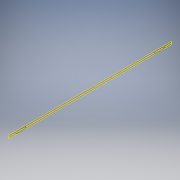
# Autodesk Inventor part: CentralLine
Saved by Autodesk Inventor 2016 (Build 200138000, 138)
## iProperties
Created: 2016-01-20
Part Number: CentralLine
Material: Generic
Document SubType Name: Modeling
Designer: KA ROSIE
Density: 1 g/cm^3
Appearance: Default
Author: KA ROSIE
Autodesk Inventor part; units mm, degrees
ref_plane "XZ Plane" through (0, 0, 0) normal (0, 1, 0) x (-1, 0, 0)
sketch "Sketch1" plane through (0, 0, 0) normal (0, 1, 0) x (-1, 0, 0)
  circle A0 centre (0, 0) radius 3
  dimension "d0" = 6
  constraints: 1 centre point, 1 coincident
  measures "d0" diameter of A0
sketch "Sketch2" plane through (0, 0, 0) normal (1, 0, 0) x (0, 1, 0)
  line L0 (0, 0) -> (-150, 0)
  ellipse E0 centre (-75, 0) end of major axis (-150, 0) minor radius 18.934
  dimension "d1" = 150
  constraints: 2 end point, 2 horizontal, 1 horizontal alignment, 1 midpoint, 2 other
  measures "d1" distance of L0.start L0.end
sketch "Sketch3" plane through (0, 0, 0) normal (0, 0, 1) x (1, 0, 0)
  circle A0 centre (0, 0) radius 3
  dimension "d2" = 6
  constraints: 1 centre point, 1 coincident
  measures "d2" diameter of A0
sweep "Sweep1" add profiles "Sketch3" path "Sketch2" path curves E0
extrude "Extrusion1" add sketch "Sketch1" along normal blind 1000
mirror "Mirror1" about plane through (0, 1000, 0) normal (0, 1, 0)
body "Solid1"
